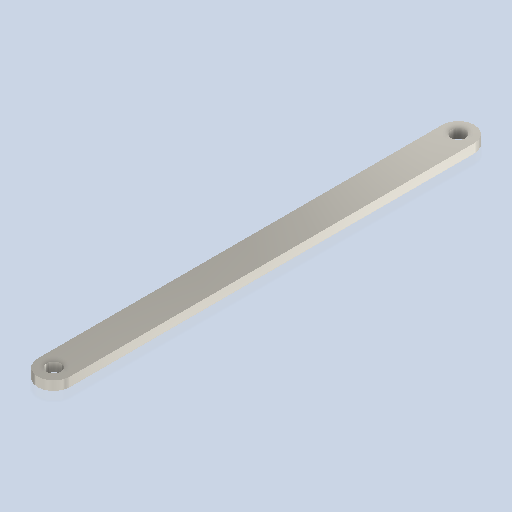
# Autodesk Inventor part: pleuelstange
Saved by Autodesk Inventor 2024.2 (Build 282272000, 272)
## iProperties
Created: 2024-04-01
Part Number: pleuelstange
Material: Titan
Document SubType Name: Modeling
Designer: Fabri
Density: 4.51 g/cm^3
Appearance: Titan
Author: Fabri
Autodesk Inventor part; units mm, degrees
ref_plane "YZ Plane" through (0, 0, 0) normal (1, 0, 0) x (0, 1, 0)
ref_plane "XZ Plane" through (0, 0, 0) normal (0, 1, 0) x (-1, 0, 0)
ref_plane "XY Plane" through (0, 0, 0) normal (0, 0, 1) x (1, 0, 0)
sketch "Skizze1" plane through (0, 0, 0) normal (0, 0, 1) x (1, 0, 0)
  line L0 (0, 0) -> (0, 44.5) construction
  line L1 (1.75, 0) -> (1.75, 44.5)
  line L2 (-1.75, 44.5) -> (-1.75, 0)
  arc A0 (-1.75, 0) -> (1.75, 0) centre (0, 0) ccw
  arc A1 (1.75, 44.5) -> (-1.75, 44.5) centre (0, 44.5) ccw
  point P0 (0, 22.25)
  dimension "d0" = 44.5
  dimension "d1" = 3.5
  constraints: 8 end point, 4 point on circle, 4 tangent, 2 centre point, 1 midpoint, 1 parallel, 1 vertical
  measures "d0" distance of L0.start L0.end
  measures "d1" distance between parallel lines of L1 L2
extrude "Extrusion1" add sketch "Skizze1" along normal blind 1
sketch "Skizze2" plane through (0, 0, 1) normal (0, 0, 1) x (1, 0, 0)
  arc A0 (1.75, 44.5) -> (-1.75, 44.5) centre (0, 44.5) ccw projected
  point P0 (0, 0)
  constraints: 1 coincident
hole "Bohrung1" at (0, 44.5, 1) at (0, 0, 1) direction (0, 0, -1) diameter 1.6 depth 1
